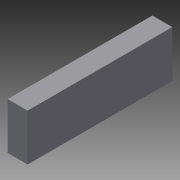
# Autodesk Inventor part: RailMount2x4_NERDS
Saved by Autodesk Inventor 2014 (Build 180170000, 170)
## iProperties
Created: 2016-01-30
Part Number: RailMount2x4_NERDS
Material: Generic
Document SubType Name: Modeling
Designer: bermudezr
Density: 1 g/cm^3
Appearance: Default
Author: bermudezr
Autodesk Inventor part; units mm, degrees
ref_plane "YZ Plane" through (0, 0, 0) normal (1, 0, 0) x (0, 1, 0)
ref_plane "XZ Plane" through (0, 0, 0) normal (0, 1, 0) x (-1, 0, 0)
ref_plane "XY Plane" through (0, 0, 0) normal (0, 0, 1) x (1, 0, 0)
sketch "Sketch1" plane through (0, 0, 0) normal (0, 0, 1) x (1, 0, 0)
  line L0 (-16.6819, 17.4202) -> (21.4181, 17.4202)
  line L1 (21.4181, 17.4202) -> (21.4181, -71.4798)
  line L2 (21.4181, -71.4798) -> (-16.6819, -71.4798)
  line L3 (-16.6819, -71.4798) -> (-16.6819, 17.4202)
  point P0 (0, 0)
  dimension "d0" = 38.1
  dimension "d1" = 88.9
  constraints: 8 end point, 2 parallel, 1 horizontal, 1 perpendicular
  measures "d0" distance of L1.end L2.end
  measures "d1" distance of L0.end L1.end
extrude "Extrusion1" add sketch "Sketch1" along normal blind 275.8186
body "Solid1"
